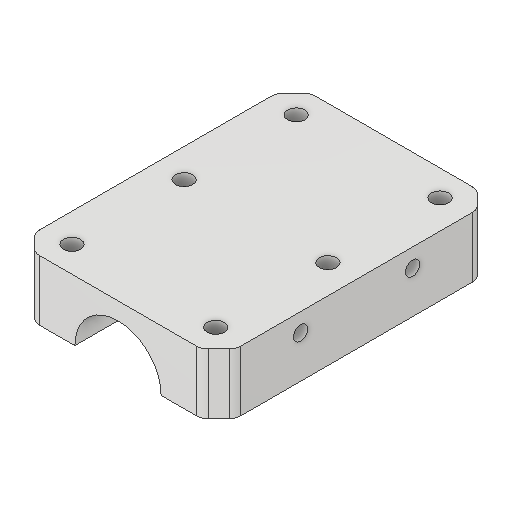
# Autodesk Inventor part: 3DP_PLA_X_end_bottom_half
Saved by Autodesk Inventor 2026.1 (Build 301233000, 233)
## iProperties
Created: 2018-07-03
Part Number: 3DP_PLA_X_end_bottom_half
Material: ABS Plastic
Document SubType Name: Modeling
Designer: Andrzej
Density: 1.06 g/cm^3
Appearance: Smooth - White
Author: Andrzej
Autodesk Inventor part; units mm, degrees
ref_plane "YZ Plane" through (0, 0, 0) normal (1, 0, 0) x (0, 1, 0)
ref_plane "XZ Plane" through (0, 0, 0) normal (0, 1, 0) x (-1, 0, 0)
ref_plane "XY Plane" through (0, 0, 0) normal (0, 0, 1) x (1, 0, 0)
sketch "Sketch1" plane through (0, 0, 0) normal (0, 0, 1) x (1, 0, 0)
  circle A0 centre (0, 0) radius 7.5
  line L0 (-17.5, 0) -> (-7.5, 0)
  line L1 (7.5, 0) -> (17.5, 0)
  line L2 (-17.5, 0) -> (-17.5, 10.5)
  line L3 (-17.5, 10.5) -> (17.5, 10.5)
  line L4 (17.5, 10.5) -> (17.5, 0)
  dimension "d5" = 15
  dimension "d6" = 0
  dimension "d8" = 0
  dimension "d11" = 10
  dimension "d13" = 10
  dimension "d19" = 10.5
  dimension "d64" = 35
  constraints: 10 end point, 3 horizontal, 2 point on circle, 1 centre point, 1 perpendicular, 1 vertical, 1 other
  measures "d5" diameter of A0
  measures "d6" distance from line of A0.centre L0
  measures "d8" distance from line of A0.centre L1
  measures "d11" distance of L0.start L0.end
  measures "d13" distance of L1.start L1.end
  measures "d19" distance from line of L3 A0.centre
  measures "d64" distance of L2.end L3.end
extrude "Extrusion1" add sketch "Sketch1" along normal blind 48 contours A0 L0 L2 L3 L4 L1
sketch "Sketch3" plane through (7.5, 0, 0) normal (0, -1, 0) x (1, 0, 0)
  line L0 (10, 0) -> (10, 48) projected
  line L1 (0, 48) -> (10, 48) projected
  line L2 (0, 0) -> (0, 48) projected
  line L3 (0, 0) -> (10, 0) projected
  line L4 (-25, 0) -> (-15, 0) projected
  line L5 (-15, 0) -> (-15, 48) projected
  line L6 (-25, 48) -> (-15, 48) projected
  line L7 (-25, 0) -> (-25, 48) projected
  point P0 (-7.5, 0)
  point P1 (5, 4.5)
  point P2 (5, 24)
  point P3 (5, 43.5)
  point P4 (-20, 43.5)
  point P5 (-20, 4.5)
  point P6 (-20, 24)
  dimension "d31" = 48
  dimension "d35" = 5
  dimension "d44" = 4.5
  dimension "d45" = 4.5
  dimension "d46" = 24
  dimension "d47" = 5
  dimension "d48" = 10
  dimension "d49" = 10
  constraints: 4 vertical alignment, 3 horizontal alignment
  measures "d31" distance between parallel lines of L3 L1
  measures "d35" distance from line of L7 point (-20, 4.5)
  measures "d44" distance from line of L4 point (-20, 4.5)
  measures "d45" distance from line of L6 point (-20, 43.5)
  measures "d46" distance from line of L4 point (-20, 24)
  measures "d47" horizontal distance of L0 point (5, 4.5)
  measures "d48" distance of L6.start L5.end
  measures "d49" distance of L1.start L0.end
hole "Hole1" at (12.5, 0, 4.5) at (12.5, 0, 24) at (12.5, 0, 43.5) at (-12.5, 0, 43.5) at (-12.5, 0, 4.5) at (-12.5, 0, 24) direction (0, 1, 0) diameter 3 end through all
chamfer "Chamfer1" distance 3 angle 45 4 edges at (17.5, 5.25, 48) (-17.5, 5.25, 48) (-17.5, 5.25, 0) (17.5, 5.25, 0)
fillet "Fillet2" radius 2 8 edges at (14.5, 5.25, 48) (17.5, 5.25, 45) (17.5, 5.25, 3) (14.5, 5.25, 0) (-14.5, 5.25, 0) (-17.5, 5.25, 3) (-17.5, 5.25, 45) (-14.5, 5.25, 48)
sketch "Sketch4" plane through (17.5, 0, 3.8284) normal (1, 0, 0) x (0, 0, -1)
  line L0 (0, 10.5) -> (-40.3431, 10.5) projected
  line L1 (3.8284, 0) -> (3.8284, 10.5) projected
  line L2 (-44.1716, 10.5) -> (-44.1716, 0) projected
  point P0 (-10.4216, 7.3)
  point P1 (-29.9216, 7.3)
  dimension "d54" = 3.2
  dimension "d55" = 14.25
  dimension "d56" = 14.25
  constraints: 1 horizontal alignment
  measures "d54" distance from line of L0 point (-10.422, 7.3)
  measures "d55" distance from line of L1 point (-10.422, 7.3)
  measures "d56" distance from line of L2 point (-29.922, 7.3)
hole "Hole2" at (17.5, 7.3, 14.25) at (17.5, 7.3, 33.75) direction (-1, 0, 0) diameter 2.5 depth 10 tip angle 118
equation "\"d13\" = d11"
equation "\"d35\" = 0.5 * d48"
equation "\"d45\" = d44"
equation "\"d46\" = 0.5 * d31"
equation "\"d47\" = d35"
equation "\"d56\" = d55"
body "Solid1"
